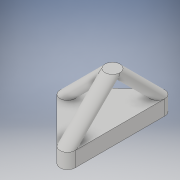
# Autodesk Inventor part: CameraTripodBaseV02
Saved by Autodesk Inventor 2018.1 (Build 221171000, 171)
## iProperties
Created: 2017-10-28
Part Number: CameraTripodBaseV02
Material: Generic
Document SubType Name: Modeling
Designer: steele
Density: 1 g/cm^3
Appearance: Default
Author: steele
Autodesk Inventor part; units mm, degrees
ref_plane "YZ Plane" through (0, 0, 0) normal (1, 0, 0) x (0, 1, 0)
ref_plane "XY Plane" through (0, 0, 0) normal (0, 0, 1) x (1, 0, 0)
sketch "Sketch2" plane through (0, 0, 0) normal (1, 0, 0) x (0, 1, 0)
  line L0 (0, 0) -> (76.2, 0) construction
  line L1 (0, 0) -> (0, -76.2) construction
  line L2 (0, 0) -> (0, 76.2) construction
  line L3 (76.2, 0) -> (0, 76.2)
  dimension "d0" = 76.2
  dimension "d1" = 76.2
  dimension "d2" = 76.2
  constraints: 8 end point, 2 vertical, 1 horizontal
  measures "d0" distance of L0.start L0.end
  measures "d1" distance of L0.start L1.end
  measures "d2" distance of L0.start L2.end
sketch "Sketch3" plane through (0, 0, 0) normal (0, 0, 1) x (1, 0, 0)
  line L0 (0, 0) -> (0, 76.2) construction
  line L1 (0, 0) -> (-76.2, 0) construction
  line L2 (0, 76.2) -> (-76.2, 0)
  dimension "d3" = 76.2
  dimension "d4" = 76.2
  constraints: 6 end point, 1 horizontal, 1 vertical
  measures "d3" distance of L0.start L0.end
  measures "d4" distance of L0.start L1.end
ref_plane "Work Plane1" through (0, 76.2, 0) normal (0, 1, 0) x (-1, 0, 0)
sketch "Sketch4" plane through (0, 76.2, 0) normal (0, 1, 0) x (-1, 0, 0)
  circle A0 centre (0, 0) radius 12.7
  dimension "d6" = 25.4
  constraints: 1 centre point, 1 coincident
  measures "d6" diameter of A0
sweep "Sweep1" add profiles "Sketch4" path "Sketch3"
sketch "Sketch5" plane through (0, 76.2, 0) normal (0, 1, 0) x (-1, 0, 0)
  circle A0 centre (0, 0) radius 12.7
  constraints: 1 centre point, 1 coincident
sweep "Sweep3" add profiles "Sketch5" path "Sketch2"
sketch "Sketch6" plane through (0, 0, 0) normal (1, 0, 0) x (0, 1, 0)
  line L0 (76.2, 8.9803) -> (76.2, -12.7) projected
  line L1 (76.2, 0) -> (0, -76.2)
  point P0 (0, 0)
  point P1 (76.2, -8.9803)
  dimension "d13" = 76.2
  constraints: 2 end point, 1 point on line
  measures "d13" distance of L1.end point (0, 0)
sketch "Sketch7" plane through (0, 76.2, 0) normal (0, 1, 0) x (-1, 0, 0)
  circle A0 centre (0, 0) radius 12.7
  constraints: 1 centre point, 1 coincident
sweep "Sweep4" add profiles "Sketch7" path "Sketch6" path curves L1
sketch "Sketch10" plane through (0, 0, 0) normal (0, 1, 0) x (-1, 0, 0)
  circle A0 centre (0, 76.2) radius 12.7 projected
  circle A1 centre (0, -76.2) radius 12.7 projected
  circle A2 centre (76.2, 0) radius 12.7 projected
  line L0 (-12.7, 76.2) -> (-12.7, -76.2)
  line L1 (6.7517, -86.9566) -> (86.5852, -7.3102)
  circle A3 centre (76.2, 0) radius 12.7 projected
  line L2 (84.8484, 9.3002) -> (8.981, 85.1796)
  point P0 (0, 0)
  constraints: 6 end point, 6 point on circle, 2 tangent, 1 vertical
extrude "Extrusion1" add sketch "Sketch10" against normal blind 25.4 contours A0 | A0 L2 A2 L1 A1 L0 | A2 L1 | A1 L1 picked at (77.9931, 4.4447) picked at (3.5769, -74.7711)
body "Solid1"
